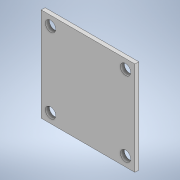
# Autodesk Inventor part: płytka
Saved by Autodesk Inventor 2020 (Build 240168000, 168)
## iProperties
Created: 2019-12-30
Part Number: płytka
Material: Ogólny
Document SubType Name: Modeling
Designer: macie
Density: 1 g/cm^3
Appearance: Domyślna
Author: macie
Autodesk Inventor part; units mm, degrees
ref_plane "YZ Plane" through (0, 0, 0) normal (1, 0, 0) x (0, 1, 0)
ref_plane "XZ Plane" through (0, 0, 0) normal (0, 1, 0) x (-1, 0, 0)
ref_plane "XY Plane" through (0, 0, 0) normal (0, 0, 1) x (1, 0, 0)
sketch "Szkic1" plane through (0, 0, 0) normal (0, 0, 1) x (1, 0, 0)
  line L0 (-16.0262, 157.75) -> (-18.2115, 157.75)
  line L1 (-18, 155.6545) -> (-18, 158.2708)
  line L2 (-16, 157.75) -> (18, 157.75)
  line L3 (18, 157.75) -> (17.9772, 121.6933)
  line L4 (17.9772, 121.6933) -> (-18.0451, 121.7161)
  line L5 (-18.0451, 121.7161) -> (-18, 157.75)
  circle A0 centre (-14.4, 154.15) radius 2
  circle A1 centre (14.4, 154.15) radius 2
  circle A2 centre (14.4, 125.35) radius 2
  circle A3 centre (-14.4, 125.35) radius 2
  line L6 (17.9772, 121.6933) -> (-18, 121.6933)
  line L7 (-18, 121.6933) -> (-18, 157.75)
  line L8 (-18, 157.75) -> (17.9772, 157.75)
  line L9 (17.9772, 157.75) -> (17.9772, 121.6933)
  circle A4 centre (-14.4, 154.15) radius 2
  circle A5 centre (14.4, 154.15) radius 2
  circle A6 centre (14.4, 125.35) radius 2
  circle A7 centre (-14.4, 125.35) radius 2
  point P0 (0, 0)
  point P1 (17.9772, 157.75)
  point P2 (-18, 121.7161)
  constraints: 20 end point, 8 centre point, 4 coincident, 4 concentric, 3 horizontal, 2 parallel, 2 perpendicular, 2 point on line
extrude "Wyciągnięcie proste1" add sketch "Szkic1" along normal blind 1.5 contours L8 L2 L9 L4 L7 L1 L0
